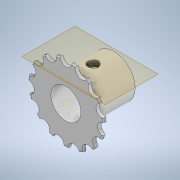
# Autodesk Inventor part: engranagem foda do beto
Saved by Autodesk Inventor 2022.1 (Build 261234020, 234B)
## iProperties
Created: 2023-09-12
Part Number: engranagem foda do beto
Material: Generic
Document SubType Name: Modeling
Designer: SENAI
Density: 1 g/cm^3
Appearance: Default
Author: SENAI
Autodesk Inventor part; units mm, degrees
ref_plane "YZ Plane" through (0, 0, 0) normal (1, 0, 0) x (0, 1, 0)
ref_plane "XY Plane" through (0, 0, 0) normal (0, 0, 1) x (1, 0, 0)
sketch "Sketch1" plane through (0, 0, 0) normal (0, 0, 1) x (1, 0, 0)
  circle A0 centre (0, 0) radius 17.5
  circle A1 centre (0, 0) radius 12.5
  arc A2 (-4.9842, 31.1032) -> (4.9842, 31.1032) centre (0, 31.5) ccw
  arc A3 (-17.2041, 26.3869) -> (-8.0975, 30.4414) centre (-12.8122, 28.7767) ccw
  arc A4 (-26.4493, 17.1081) -> (-19.7791, 24.5161) centre (-23.4091, 21.0776) ccw
  arc A5 (-31.1211, 4.8711) -> (-28.0407, 14.3517) centre (-29.9583, 9.734) ccw
  arc A6 (-30.4118, -8.2081) -> (-31.4538, 1.7058) centre (-31.3274, -3.2926) ccw
  arc A7 (-24.444, -19.8681) -> (-29.4283, -11.2351) centre (-27.2798, -15.75) ccw
  arc A8 (-14.2497, -28.0927) -> (-22.3143, -22.2333) centre (-18.5152, -25.484) ccw
  arc A9 (-1.5914, -31.4598) -> (-11.342, -29.3872) centre (-6.5492, -30.8116) ccw
  arc A10 (11.342, -29.3872) -> (1.5914, -31.4598) centre (6.5492, -30.8116) ccw
  arc A11 (22.3143, -22.2333) -> (14.2497, -28.0927) centre (18.5152, -25.484) ccw
  arc A12 (29.4283, -11.2351) -> (24.444, -19.8681) centre (27.2798, -15.75) ccw
  arc A13 (31.4538, 1.7058) -> (30.4118, -8.2081) centre (31.3274, -3.2926) ccw
  arc A14 (28.0407, 14.3517) -> (31.1211, 4.8711) centre (29.9583, 9.734) ccw
  arc A15 (19.7791, 24.5161) -> (26.4493, 17.1081) centre (23.4091, 21.0776) ccw
  arc A16 (8.0975, 30.4414) -> (17.2041, 26.3869) centre (12.8122, 28.7767) ccw
  arc A17 (8.0975, 30.4414) -> (4.9842, 31.1032) centre (0, 0) ccw
  arc A18 (19.7791, 24.5161) -> (17.2041, 26.3869) centre (0, 0) ccw
  arc A19 (28.0407, 14.3517) -> (26.4493, 17.1081) centre (0, 0) ccw
  arc A20 (31.4538, 1.7058) -> (31.1211, 4.8711) centre (0, 0) ccw
  arc A21 (29.4283, -11.2351) -> (30.4118, -8.2081) centre (0, 0) ccw
  arc A22 (22.3143, -22.2333) -> (24.444, -19.8681) centre (0, 0) ccw
  arc A23 (11.342, -29.3872) -> (14.2497, -28.0927) centre (0, 0) ccw
  arc A24 (-1.5914, -31.4598) -> (1.5914, -31.4598) centre (0, 0) ccw
  arc A25 (-14.2497, -28.0927) -> (-11.342, -29.3872) centre (0, 0) ccw
  arc A26 (-24.444, -19.8681) -> (-22.3143, -22.2333) centre (0, 0) ccw
  arc A27 (-30.4118, -8.2081) -> (-29.4283, -11.2351) centre (0, 0) ccw
  arc A28 (-31.1211, 4.8711) -> (-31.4538, 1.7058) centre (0, 0) ccw
  arc A29 (-4.9842, 31.1032) -> (-19.7791, 24.5161) centre (0, 0) ccw
  arc A30 (-26.4493, 17.1081) -> (-28.0407, 14.3517) centre (0, 0) ccw
  point P0 (-8.0975, 30.4414)
  point P1 (-17.2041, 26.3869)
  dimension "d1" = 35
  dimension "d2" = 25
  dimension "d3" = 10
  dimension "d6" = 360
  constraints: 58 point on circle, 31 centre point, 3 coincident, 61 other
  measures "d1" diameter of A0
  measures "d2" diameter of A1
  measures "d3" diameter of A2
extrude "Extrusion1" add sketch "Sketch1" along normal blind 2.8 contours A2 A17 A16 A18 A15 A19 A14 A20 A13 A21 A12 A22 A11 A23 A10 A24 A9 A25 A8 A26 A7 A27 A6 A28 A5 A30 A4 A29 A3
sketch "Sketch2" plane through (0, 0, 2.8) normal (0, 0, 1) x (1, 0, 0)
  point P0 (0, 0)
fillet "Fillet1" radius 1 30 edges at (6.5492, 30.8116, 2.8) (6.5492, 30.8116, 0) (-6.5492, 30.8116, 2.8) (-6.5492, 30.8116, 0) (-18.5152, 25.484, 2.8) (-18.5152, 25.484, 0) (18.5152, 25.484, 2.8) (18.5152, 25.484, 0) (27.2798, 15.75, 2.8) (27.2798, 15.75, 0) (-27.2798, 15.75, 2.8) (-27.2798, 15.75, 0) (31.3274, 3.2926, 2.8) (31.3274, 3.2926, 0) (29.9583, -9.734, 2.8) (29.9583, -9.734, 0) (23.4091, -21.0776, 2.8) (23.4091, -21.0776, 0) (12.8122, -28.7767, 2.8) (12.8122, -28.7767, 0) (0, -31.5, 2.8) (0, -31.5, 0) (-12.8122, -28.7767, 2.8) (-12.8122, -28.7767, 0) (-23.4091, -21.0776, 2.8) (-23.4091, -21.0776, 0) (-29.9583, -9.734, 2.8) (-29.9583, -9.734, 0) (-31.3274, 3.2926, 2.8) (-31.3274, 3.2926, 0)
sketch "Sketch3" plane through (0, 0, 2.8) normal (0, 0, 1) x (1, 0, 0)
  circle A0 centre (0, 0) radius 17.5
  circle A1 centre (0, 0) radius 12.5
  dimension "d11" = 35
  dimension "d12" = 25
  constraints: 2 centre point, 2 coincident
  measures "d11" diameter of A0
  measures "d12" diameter of A1
extrude "Extrusion2" add sketch "Sketch3" against normal blind 40 contours A0 | A1
sketch "Sketch4" plane through (0, 0, 2.8) normal (0, 0, 1) x (1, 0, 0)
  circle A0 centre (0, 0) radius 12.5
  dimension "d15" = 25
  constraints: 1 centre point, 1 coincident
  measures "d15" diameter of A0
extrude "Extrusion3" cut sketch "Sketch4" against normal blind 40
ref_plane "Work Plane1" through (0, 17.5, 0) normal (0, 1, 0) x (-1, 0, 0)
sketch "Sketch5" plane through (0, 17.5, 0) normal (0, 1, 0) x (-1, 0, 0)
  circle A0 centre (0, -19.656) radius 4.275
  point P0 (0, 0)
  dimension "d19" = 8.55
  constraints: 1 centre point
  measures "d19" diameter of A0
hole "Hole1" at (0, 17.5, -19.656) direction (0, -1, 0) diameter 8.55 depth 8 tip angle 118
thread "Thread1" size "M10x1.5" class "6H" standard "ISO Metric profile" full length
body "Solid1"
